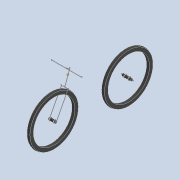
# Autodesk Inventor part: LW sketch
Saved by Autodesk Inventor 2021 (Build 250183000, 183)
## iProperties
Created: 2020-05-07
Part Number: LW sketch
Material: Generic
Document SubType Name: Modeling
Designer: Hannah
Appearance: Default
Surface Area: 8694.89 cm^2
Volume: 10910.6 cm^3
Author: Hannah
Autodesk Inventor part; units mm, degrees
ref_plane "Work Plane6" through (84.6427, 87.4734, -400.3058) normal (-1, 0, 0) x (0, 0.9396926, -0.3420201)
ref_plane "Work Plane5" through (-84.6427, 83.5886, -432.9589) normal (1, 0, 0) x (0, -0.9396926, 0.3420201)
ref_plane "Work Plane6" through (84.6427, 87.4734, -400.3058) normal (-1, 0, 0) x (0, 0.9396926, -0.3420201)
ref_plane "Work Plane3" through (-84.6427, 60, -486.347) normal (0, 1, 0) x (-1, 0, 0)
ref_plane "Work Plane1" through (-84.6427, 60, -486.347) normal (0, 0, 1) x (1, 0, 0)
ref_plane "Work Plane2" through (0, 0, 618) normal (0, 0, 1) x (1, 0, 0)
ref_plane "Work Plane4" through (-84.6427, -310, -486.347) normal (0, 1, 0) x (-1, 0, 0)
sketch3d "FEA outline"
sketch "Sketch4" plane through (0, 0, 0) normal (1, 0, 0) x (0, 1, 0)
  line L0 (1144.2962, 185.3262) -> (-521.8385, 791.7497) projected
  line L1 (60, 633.1867) -> (42.899, 586.202)
  point P0 (0, 0)
  point P1 (60, -486.347)
  dimension "d64" = 50
  constraints: 2 end point, 1 perpendicular, 1 point on line, 1 vertical alignment
  measures "d64" distance of L1.start L1.end
sketch3d "placeholders"
ref_plane "Work Plane7" through (50, 60, 633.1867) normal (0, 0, 1) x (1, 0, 0)
sketch "Sketch2" plane through (50, 60, 633.1867) normal (0, 0, 1) x (1, 0, 0)
  line L0 (-72, -311) -> (-28, -311)
  line L1 (-28, -311) -> (-28, -363.4066)
  line L2 (-72, -363.4066) -> (-72, -311)
  line L3 (-100, 0) -> (0, 0) projected
  arc A0 (-72, -363.4066) -> (-28, -363.4066) centre (-50, -330) ccw
  line L4 (0, -17.5) -> (0, 0)
  line L5 (0, 0) -> (-100, 0)
  line L6 (-100, 0) -> (-100, -17.5)
  line L7 (-82, -25) -> (-80, -25)
  line L8 (-80, -25) -> (-80, -17.5)
  line L9 (-82, -17.5) -> (-82, -25)
  line L10 (-20, -25) -> (-18, -25)
  line L11 (-18, -25) -> (-18, -17.5)
  line L12 (-20, -17.5) -> (-20, -25)
  line L13 (-100, -17.5) -> (-82, -17.5)
  line L14 (-80, -17.5) -> (-20, -17.5)
  line L15 (-18, -17.5) -> (0, -17.5)
  point P0 (-50, -60)
  point P1 (-50, -311)
  point P2 (-50, -17.5)
  point P3 (-100, 0)
  point P4 (-50, -17.5)
  point P5 (-50, 0)
  dimension "TyreWidth" = 44
  dimension "d24" = 40
  dimension "BSD" = 622
  dimension "d26" = 660
  dimension "FrontHubSpacing" = 100
  dimension "d30" = 60
  dimension "d31" = 2
  dimension "d32" = 50
  dimension "d33" = 35
  constraints: 30 end point, 7 parallel, 6 horizontal, 6 perpendicular, 4 midpoint, 4 vertical alignment, 2 collinear, 2 equal length, 2 point on circle, 2 point on line, 1 centre point
  measures "TyreWidth" distance between parallel lines of L1 L2
  measures "d24" radius of A0
  measures "BSD" diameter of L0 L3
  measures "d26" diameter of A0.centre L3
  measures "FrontHubSpacing" distance of L6.end L4.start
  measures "d30" distance between parallel lines of L12 L8
  measures "d31" distance of L10.start L10.end
  measures "d32" diameter of L7 L3
  measures "d33" diameter of L13 L3
revolve "Revolution1" add sketch "Sketch2" angle 360 about axis through (-50, 60, 633.1867) along (1, 0, 0)
ref_plane "Work Plane8" through (84.6427, 60, -486.347) normal (0, 0, 1) x (1, 0, 0)
sketch "Sketch3" plane through (84.6427, 255, -486.347) normal (0, 0, 1) x (1, 0, 0)
  line L0 (-106.6427, -506) -> (-62.6427, -506)
  line L1 (-62.6427, -506) -> (-62.6427, -558.4066)
  line L2 (-106.6427, -558.4066) -> (-106.6427, -506)
  line L3 (-37.8915, -195) -> (62.1085, -195)
  arc A0 (-106.6427, -558.4066) -> (-62.6427, -558.4066) centre (-84.6427, -525) ccw
  line L4 (-17.1427, -212.5) -> (-17.1427, -195)
  line L5 (-17.1427, -195) -> (-152.1427, -195)
  line L6 (-152.1427, -195) -> (-152.1427, -212.5)
  line L7 (-116.6427, -220) -> (-114.6427, -220)
  line L8 (-114.6427, -220) -> (-114.6427, -212.5)
  line L9 (-116.6427, -212.5) -> (-116.6427, -220)
  line L10 (-54.6427, -220) -> (-52.6427, -220)
  line L11 (-52.6427, -220) -> (-52.6427, -212.5)
  line L12 (-54.6427, -212.5) -> (-54.6427, -220)
  line L13 (-152.1427, -212.5) -> (-116.6427, -212.5)
  line L14 (-114.6427, -212.5) -> (-54.6427, -212.5)
  line L15 (-52.6427, -212.5) -> (-17.1427, -212.5)
  line L16 (-169.2853, -195) -> (0, -195) projected
  point P0 (-84.6427, -506)
  point P1 (-50, 0)
  point P2 (-84.6427, -212.5)
  point P3 (-84.6427, -195)
  point P4 (-84.6427, -255)
  dimension "d41" = 44
  dimension "d39" = 40
  dimension "d42" = 622
  dimension "d40" = 660
  dimension "RearHubWidth" = 135
  dimension "d35" = 60
  dimension "d36" = 2
  dimension "d37" = 50
  dimension "d34" = 35
  constraints: 32 end point, 7 parallel, 6 horizontal, 6 perpendicular, 3 collinear, 3 midpoint, 3 vertical alignment, 2 equal length, 2 point on circle, 2 point on line, 1 centre point
  measures "d41" distance between parallel lines of L1 L2
  measures "d39" radius of A0
  measures "d42" diameter of L0 L3
  measures "d40" diameter of A0.centre L3
  measures "RearHubWidth" distance of L6.end L4.start
  measures "d35" distance between parallel lines of L12 L8
  measures "d36" distance of L10.start L10.end
  measures "d37" diameter of L7 L3
  measures "d34" diameter of L13 L3
revolve "Revolution2" add sketch "Sketch3" angle 360 about axis through (46.7512, 60, -486.347) along (1, 0, 0)
equation "\"d3\" = d2"
equation "\"d4\" = d2"
equation "\"d18\" = d17"
equation "\"d26\" = tyreOD - 2 * d24"
equation "\"d41\" = TyreWidth"
equation "\"d42\" = BSD"
equation "\"d40\" = tyreOD - 2 * d39"
equation "\"d2\" = 60"
equation "\"d17\" = 25"
equation "\"tyreOD\" = 740"
body "Solid1"
